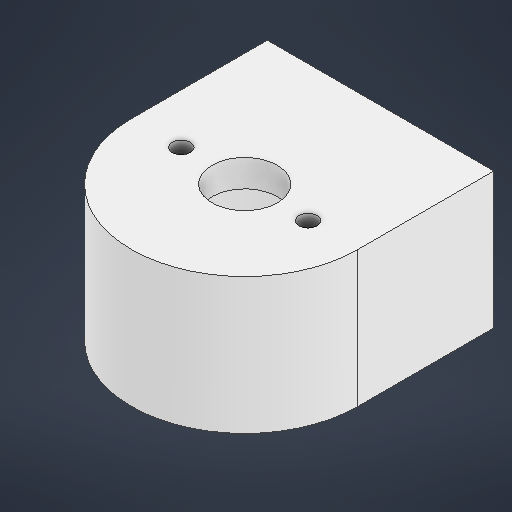
# Autodesk Inventor part: Dribbler motor mount lower section
Saved by Autodesk Inventor 2026.1 (Build 301233000, 233)
## iProperties
Created: 2025-12-08
Part Number: Dribbler motor mount lower section
Material: Generisch
Document SubType Name: Modeling
Designer: Familie
Density: 1 g/cm^3
Appearance: Weiß
Author: Familie
Autodesk Inventor part; units mm, degrees
ref_plane "YZ Plane" through (0, 0, 0) normal (1, 0, 0) x (0, 1, 0)
ref_plane "XZ Plane" through (0, 0, 0) normal (0, 1, 0) x (-1, 0, 0)
ref_plane "XY Plane" through (0, 0, 0) normal (0, 0, 1) x (1, 0, 0)
sketch "Skizze1" plane through (0, 0, 0) normal (0, 0, 1) x (1, 0, 0)
  circle A0 centre (0, 0) radius 10.1
  circle A1 centre (0, 0) radius 12.5
  circle A2 centre (-7, 0) radius 1
  circle A3 centre (7, 0) radius 1
  circle A4 centre (0, 0) radius 3.6
  line L0 (-12.5, 0) -> (-12.5, 15)
  line L1 (-12.5, 15) -> (12.5, 15)
  line L2 (12.5, 15) -> (12.5, 0)
  dimension "d0" = 20.2
  dimension "d1" = 25
  dimension "d2" = 2
  dimension "d3" = 2
  dimension "d4" = 7.2
  dimension "d5" = 7
  dimension "d6" = 7
  dimension "d11" = 15
  constraints: 6 end point, 5 centre point, 3 coincident, 2 horizontal alignment, 2 point on circle, 2 tangent, 1 parallel, 1 perpendicular, 1 vertical, 1 vertical alignment
  measures "d0" diameter of A0
  measures "d1" diameter of A1
  measures "d2" diameter of A3
  measures "d3" diameter of A2
  measures "d4" diameter of A4
  measures "d5" distance of point (0, 0) A2.centre
  measures "d6" distance of point (0, 0) A3.centre
  measures "d11" distance of L1.end L2.end
extrude "Extrusion1" add sketch "Skizze1" against normal blind 15 contours A1 | A1 L0 L1 L2
extrude "Extrusion2" add sketch "Skizze1" against normal blind 3 contours A0
